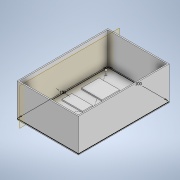
# Autodesk Inventor part: chestbox
Saved by Autodesk Inventor 2021 (Build 250183000, 183)
## iProperties
Created: 2021-12-03
Part Number: chestbox
Material: Generic
Document SubType Name: Modeling
Designer: Marcin
Density: 1 g/cm^3
Appearance: Default
Author: Marcin
Autodesk Inventor part; units mm, degrees
ref_plane "XZ Plane" through (0, 0, 0) normal (0, 1, 0) x (-1, 0, 0)
ref_plane "XY Plane" through (0, 0, 0) normal (0, 0, 1) x (1, 0, 0)
sketch "Sketch1" plane through (0, 0, 0) normal (0, 1, 0) x (-1, 0, 0)
  line L0 (-50, 75) -> (50, 75)
  line L1 (50, 75) -> (50, -75)
  line L2 (50, -75) -> (-50, -75)
  line L3 (-50, -75) -> (-50, 75)
  line L4 (-50, 75) -> (50, -75) construction
  line L5 (50, 75) -> (-50, -75) construction
  line L6 (52, -77) -> (52, 77)
  line L7 (52, 77) -> (-52, 77)
  line L8 (-52, 77) -> (-52, -77)
  line L9 (-52, -77) -> (52, -77)
  point P0 (0, 0)
  dimension "d0" = 100
  dimension "d1" = 150
  dimension "d2" = 2
  constraints: 20 end point, 4 parallel, 2 midpoint, 2 perpendicular, 1 horizontal, 3 other
  measures "d0" distance of L1.end L2.end
  measures "d1" distance of L0.end L1.end
  measures "d2" distance between parallel lines of L1 L6
extrude "Extrusion1" add sketch "Sketch1" along normal blind 55
extrude "Extrusion2" add sketch "Sketch1" against normal blind 2 contours L0 L1 L2 L3 | L9 L8 L7 L6
sketch "Sketch2" plane through (0, 0, 0) normal (0, 1, 0) x (1, 0, 0)
  point P0 (0, 0)
ref_plane "Work Plane1" through (-40, 0, 0) normal (1, 0, 0) x (0, 1, 0)
sketch "Sketch4" plane through (-40, 0, 0) normal (1, 0, 0) x (0, 1, 0)
  line L0 (-22.2589, -61.7044) -> (45.831, -61.7044)
  line L1 (0, 75) -> (0, -75) projected
  line L2 (0, -63.0544) -> (7, -63.0544)
  line L3 (7, -63.0544) -> (7, -63.5044)
  arc A0 (7, -63.5044) -> (8.8, -61.7044) centre (7, -61.7044) ccw
  line L4 (8.8, -61.7044) -> (0, -61.7044)
  line L5 (0, -63.0544) -> (0, -61.7044)
  point P0 (0, 0)
  dimension "d9" = 2.7
  dimension "d10" = 3.6
  dimension "d11" = 7
  constraints: 10 end point, 5 point on line, 2 perpendicular, 2 point on circle, 1 centre point, 1 collinear, 1 horizontal
  measures "d9" diameter of L2 L0
  measures "d10" diameter of L3.end L0
  measures "d11" distance from line of L1 L2.end
revolve "Revolution1" add sketch "Sketch4" angle 360 about axis through (-40, -22.2589, -61.7044) along (0, 1, 0)
sketch "Sketch6" plane through (0, 0, 0) normal (0, 1, 0) x (1, 0, 0)
  line L0 (-40, 50) -> (-5, 50)
  line L1 (-5, 50) -> (-5, 20)
  line L2 (-5, 20) -> (-40, 20)
  line L3 (-40, 20) -> (-40, 50)
  line L4 (-50, 75) -> (50, 75) projected
  line L5 (-50, -75) -> (-50, 75) projected
  line L6 (-40, 4) -> (-5, 4)
  line L7 (-5, 4) -> (-5, -13)
  line L8 (-5, -13) -> (-40, -13)
  line L9 (-40, -13) -> (-40, 4)
  point P0 (0, 0)
  dimension "d15" = 35
  dimension "d16" = 30
  dimension "d17" = 25
  dimension "d18" = 10
  dimension "d21" = 71
  dimension "d22" = 17
  constraints: 16 end point, 5 parallel, 2 horizontal, 2 perpendicular, 1 collinear
  measures "d15" distance of L1.end L2.end
  measures "d16" distance of L0.end L1.end
  measures "d17" distance between parallel lines of L4 L0
  measures "d18" distance between parallel lines of L5 L3
  measures "d21" distance between parallel lines of L4 L6
  measures "d22" distance of L8.end L6.start
extrude "Extrusion3" add sketch "Sketch6" along normal blind 2
body "Solid1"
